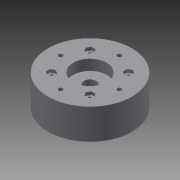
# Autodesk Inventor part: bowl
Saved by Autodesk Inventor 2014 (Build 180170000, 170)
## iProperties
Created: 2014-01-13
Part Number: bowl
Material: Générique
Document SubType Name: Modeling
Designer: helly
Density: 1 g/cm^3
Appearance: Par défaut
Author: helly
Autodesk Inventor part; units mm, degrees
ref_plane "YZ Plane" through (0, 0, 0) normal (1, 0, 0) x (0, 1, 0)
ref_plane "XZ Plane" through (0, 0, 0) normal (0, 1, 0) x (-1, 0, 0)
ref_plane "XY Plane" through (0, 0, 0) normal (0, 0, 1) x (1, 0, 0)
sketch "Esquisse1" plane through (0, 0, 0) normal (0, 0, 1) x (1, 0, 0)
  circle A0 centre (0, 0) radius 40
  circle A1 centre (0, 0) radius 6
  line L0 (0, 0) -> (16, 0) construction
  circle A2 centre (0, 0) radius 16 construction
  line L1 (6, 0) -> (16, 0) construction
  line L2 (0, 0) -> (0, 28) construction
  circle A3 centre (0, 28) radius 2
  circle A4 centre (-28, 0) radius 2
  circle A5 centre (0, -28) radius 2
  circle A6 centre (28, 0) radius 2
  dimension "d1" = 12
  dimension "d0" = 80
  dimension "d3" = 10
  dimension "d5" = 4
  dimension "d6" = 28
  dimension "d9" = 360
  constraints: 9 coincident, 6 end point, 5 centre point, 2 horizontal alignment, 1 collinear, 1 horizontal, 1 perpendicular, 1 point on line, 19 other
  measures "d0" diameter of A0
  measures "d3" distance of L1.start L0.end
  measures "d5" diameter of A3
  measures "d6" distance of L2.start L2.end
extrude "Extrusion1" add sketch "Esquisse1" along normal blind 29
sketch "Esquisse2" plane through (0, 0, 29) normal (0, 0, 1) x (1, 0, 0)
  circle A0 centre (0, 0) radius 6 projected
  circle A1 centre (0, 0) radius 40 projected
  line L0 (0, 0) -> (6, 0) construction
  line L1 (6, 0) -> (16, 0) construction
  circle A2 centre (0, 0) radius 16
  dimension "d15" = 10
  constraints: 4 end point, 2 horizontal alignment, 1 coincident, 1 collinear, 1 horizontal, 3 other
  measures "d15" distance of L0.end L1.end
extrude "Extrusion2" cut sketch "Esquisse2" against normal blind 10 contours A2
sketch "Esquisse3" plane through (0, 0, 0) normal (0, 0, -1) x (-1, 0, 0)
  circle A0 centre (0, 0) radius 6 projected
  circle A1 centre (-28, 0) radius 2 projected
  circle A2 centre (0, -28) radius 2 projected
  circle A3 centre (28, 0) radius 2 projected
  circle A4 centre (0, 28) radius 2 projected
  circle A5 centre (0, 0) radius 40 projected
  line L0 (3.5, 25.9793) -> (0, 23.9585)
  line L1 (0, 23.9585) -> (-3.5, 25.9793)
  line L2 (-3.5, 25.9793) -> (-3.5, 30.0207)
  line L3 (-3.5, 30.0207) -> (0, 32.0415)
  line L4 (0, 32.0415) -> (3.5, 30.0207)
  line L5 (3.5, 30.0207) -> (3.5, 25.9793)
  line L6 (-3.5, 25.9793) -> (3.5, 25.9793) construction
  line L7 (0, 0) -> (0, -40) construction
  line L8 (-25.9793, 3.5) -> (-23.9585, 0)
  line L9 (-23.9585, 0) -> (-25.9793, -3.5)
  line L10 (-25.9793, -3.5) -> (-30.0207, -3.5)
  line L11 (-30.0207, -3.5) -> (-32.0415, 0)
  line L12 (-32.0415, 0) -> (-30.0207, 3.5)
  line L13 (-30.0207, 3.5) -> (-25.9793, 3.5)
  line L14 (-3.5, -25.9793) -> (0, -23.9585)
  line L15 (0, -23.9585) -> (3.5, -25.9793)
  line L16 (3.5, -25.9793) -> (3.5, -30.0207)
  line L17 (3.5, -30.0207) -> (0, -32.0415)
  line L18 (0, -32.0415) -> (-3.5, -30.0207)
  line L19 (-3.5, -30.0207) -> (-3.5, -25.9793)
  line L20 (25.9793, -3.5) -> (23.9585, 0)
  line L21 (23.9585, 0) -> (25.9793, 3.5)
  line L22 (25.9793, 3.5) -> (30.0207, 3.5)
  line L23 (30.0207, 3.5) -> (32.0415, 0)
  line L24 (32.0415, 0) -> (30.0207, -3.5)
  line L25 (30.0207, -3.5) -> (25.9793, -3.5)
  point P0 (-25.9793, 3.5)
  point P1 (-3.5, -25.9793)
  point P2 (25.9793, -3.5)
  dimension "d18" = 7
  dimension "d21" = 360
  constraints: 52 end point, 4 point on line, 1 coincident, 1 parallel, 1 perpendicular, 1 vertical, 1 vertical alignment, 67 other
  measures "d18" distance of L1.end L6.end
extrude "Extrusion3" cut sketch "Esquisse3" against normal blind 3 contours L0 L1 L2 L3 L4 L5 | L8 L9 L10 L11 L12 L13 | L14 L15 L16 L17 L18 L19 | L20 L21 L22 L23 L24 L25
sketch "Esquisse4" plane through (0, 0, 29) normal (0, 0, 1) x (1, 0, 0)
  circle A0 centre (0, 0) radius 16 projected
  circle A1 centre (0, 0) radius 40 projected
  line L0 (0, 0) -> (18.3848, 18.3848) construction
  line L1 (0, 0) -> (26, 0) construction
  circle A2 centre (18.3848, 18.3848) radius 2
  circle A3 centre (-18.3848, 18.3848) radius 2
  circle A4 centre (-18.3848, -18.3848) radius 2
  circle A5 centre (18.3848, -18.3848) radius 2
  dimension "d25" = 26
  dimension "d26" = 45
  dimension "d27" = 4
  dimension "d30" = 360
  constraints: 4 centre point, 4 end point, 1 coincident, 1 equal length, 1 horizontal, 1 point on line, 9 other
  measures "d25" distance of L0.start L0.end
  measures "d26" angle of L1 L0
  measures "d27" diameter of A2
extrude "Extrusion4" cut sketch "Esquisse4" against normal through all contours A2 | A3 | A4 | A5
sketch "Esquisse5" plane through (0, 0, 29) normal (0, 0, 1) x (1, 0, 0)
  circle A0 centre (-18.3848, -18.3848) radius 2 projected
  circle A1 centre (18.3848, 18.3848) radius 2 projected
  circle A2 centre (-18.3848, 18.3848) radius 2 projected
  circle A3 centre (18.3848, -18.3848) radius 2 projected
  circle A4 centre (0, 0) radius 16 projected
  circle A5 centre (0, 0) radius 40 projected
  line L0 (14.8848, 16.3641) -> (14.8848, 20.4055)
  line L1 (14.8848, 20.4055) -> (18.3848, 22.4262)
  line L2 (18.3848, 22.4262) -> (21.8848, 20.4055)
  line L3 (21.8848, 20.4055) -> (21.8848, 16.3641)
  line L4 (21.8848, 16.3641) -> (18.3848, 14.3433)
  line L5 (18.3848, 14.3433) -> (14.8848, 16.3641)
  line L6 (0, 0) -> (0, 40) construction
  line L7 (14.8848, 16.3641) -> (21.8848, 16.3641) construction
  line L8 (-16.3641, 14.8848) -> (-20.4055, 14.8848)
  line L9 (-20.4055, 14.8848) -> (-22.4262, 18.3848)
  line L10 (-22.4262, 18.3848) -> (-20.4055, 21.8848)
  line L11 (-20.4055, 21.8848) -> (-16.3641, 21.8848)
  line L12 (-16.3641, 21.8848) -> (-14.3433, 18.3848)
  line L13 (-14.3433, 18.3848) -> (-16.3641, 14.8848)
  line L14 (-14.8848, -16.3641) -> (-14.8848, -20.4055)
  line L15 (-14.8848, -20.4055) -> (-18.3848, -22.4262)
  line L16 (-18.3848, -22.4262) -> (-21.8848, -20.4055)
  line L17 (-21.8848, -20.4055) -> (-21.8848, -16.3641)
  line L18 (-21.8848, -16.3641) -> (-18.3848, -14.3433)
  line L19 (-18.3848, -14.3433) -> (-14.8848, -16.3641)
  line L20 (16.3641, -14.8848) -> (20.4055, -14.8848)
  line L21 (20.4055, -14.8848) -> (22.4262, -18.3848)
  line L22 (22.4262, -18.3848) -> (20.4055, -21.8848)
  line L23 (20.4055, -21.8848) -> (16.3641, -21.8848)
  line L24 (16.3641, -21.8848) -> (14.3433, -18.3848)
  line L25 (14.3433, -18.3848) -> (16.3641, -14.8848)
  dimension "d34" = 7
  dimension "d37" = 360
  constraints: 52 end point, 1 coincident, 1 parallel, 1 perpendicular, 1 vertical, 1 vertical alignment, 63 other
  measures "d34" distance of L0.start L3.end
extrude "Extrusion5" cut sketch "Esquisse5" against normal blind 3 contours L0 L1 L2 L3 L4 L5 | L8 L9 L10 L11 L12 L13 | L14 L15 L16 L17 L18 L19 | L20 L21 L22 L23 L24 L25
